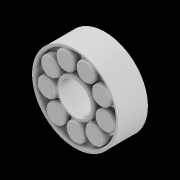
# Autodesk Inventor part: PIP-KL_parametriserad_02
Saved by Autodesk Inventor 2020 (Build 240168000, 168)
## iProperties
Created: 2020-11-21
Part Number: PIP-KL_parametriserad_02
Material: Generic
Document SubType Name: Modeling
Designer: Gottfrid
Density: 1 g/cm^3
Appearance: Default
Author: Gottfrid
Autodesk Inventor part; units mm, degrees
ref_plane "YZ Plane" through (0, 0, 0) normal (1, 0, 0) x (0, 1, 0)
ref_plane "XZ Plane" through (0, 0, 0) normal (0, 1, 0) x (-1, 0, 0)
ref_plane "XY Plane" through (0, 0, 0) normal (0, 0, 1) x (1, 0, 0)
sketch "Sketch1" plane through (0, 0, 0) normal (0, 0, 1) x (1, 0, 0)
  circle A0 centre (0, 0) radius 4
  circle A1 centre (0, 0) radius 4.75
  circle A2 centre (0, 0) radius 10
  circle A3 centre (0, 0) radius 10.75
  circle A4 centre (0, -7.375) radius 2.375
  dimension "d0" = 8
  dimension "d1" = 9.5
  dimension "d2" = 20
  dimension "d3" = 21.5
  dimension "d4" = 7.375
  dimension "d5" = 4.75
  constraints: 5 centre point, 4 coincident, 1 vertical alignment
  measures "d0" diameter of A0
  measures "d1" diameter of A1
  measures "d2" diameter of A2
  measures "d3" diameter of A3
  measures "d4" distance of A4.centre point (0, 0)
  measures "d5" diameter of A4
extrude "Extrusion1" add sketch "Sketch1" along normal blind 1.5 contours A0 | A1
extrude "Extrusion8" add sketch "Sketch1" along normal blind 1.5 contours A4
extrude "Extrusion9" add sketch "Sketch1" along normal blind 1.5 contours A3
sketch "Sketch17" plane through (0, 0, 1.5) normal (0, 0, 1) x (1, 0, 0)
  circle A0 centre (0, 0) radius 4.75 projected
extrude "Extrusion10" add sketch "Sketch17" along normal blind 1.5 draft 35
sketch "Sketch18" plane through (0, -7.375, 1.5) normal (0, 0, 1) x (1, 0, 0)
  circle A0 centre (0, 0) radius 2.375 projected
  point P0 (0, 7.375)
extrude "Extrusion11" add sketch "Sketch18" along normal blind 1.5 draft -35
sketch "Sketch19" plane through (0, 0, 1.5) normal (0, 0, 1) x (1, 0, 0)
  circle A0 centre (0, 0) radius 10 projected
  circle A1 centre (0, 0) radius 10.75 projected
extrude "Extrusion12" add sketch "Sketch19" along normal blind 1.5 draft 35
sketch "Sketch20" plane through (0, 0, 3) normal (0, 0, 1) x (1, 0, 0)
  circle A0 centre (0, 0) radius 5.8003 projected
extrude "Extrusion13" add sketch "Sketch20" along normal blind 0.75
sketch "Sketch21" plane through (0, -7.375, 3) normal (0, 0, 1) x (1, 0, 0)
  circle A0 centre (0, 0) radius 1.3247 projected
  point P0 (0, 7.375)
extrude "Extrusion14" add sketch "Sketch21" along normal blind 0.75
sketch "Sketch22" plane through (0, 0, 3) normal (0, 0, 1) x (1, 0, 0)
  circle A0 centre (0, 0) radius 8.9497 projected
  circle A1 centre (0, 0) radius 11.8003 projected
extrude "Extrusion15" add sketch "Sketch22" along normal blind 0.75
chamfer "Chamfer2" distance 0.3 angle 45 3 edges at (-10, 0, 0) (-2.375, -7.375, 0) (-4.75, 0, 0)
mirror "Mirror1" about plane through (0, 0, 3.75) normal (0, 0, 1) of "Extrusion13", "Extrusion10", "Extrusion1"
mirror "Mirror2" about plane through (0, -7.375, 3.75) normal (0, 0, 1) of "Extrusion8", "Extrusion11", "Extrusion14"
mirror "Mirror3" about plane through (0, 0, 3.75) normal (0, 0, 1) of "Extrusion9", "Extrusion12", "Extrusion15"
extrude "Extrusion16" cut sketch "Sketch1" along normal blind 99999 contours A0
extrude "Extrusion17" cut sketch "Sketch1" along normal blind 99999 contours A0 | A1 | A2 | A3 | A4 keep common part
chamfer "Chamfer3" distance 0.3 angle 45 3 edges at (-10, 0, 7.5) (-2.375, -7.375, 7.5) (-4.75, 0, 7.5)
pattern_circular "Circular Pattern2" count 9 over 360 about axis through (0, 0, 0) along (0, 0, 1) of "Extrusion8", "Extrusion11", "Extrusion14", "Mirror2"
chamfer "Chamfer4" distance 0.3 angle 45 14 edges at (-7.6754, 1.0583, 7.5) (-5.1994, 5.7443, 7.5) (-0.2906, 7.7425, 7.5) (4.7542, 6.1179, 7.5) (7.5744, 1.6307, 7.5) (6.8505, -3.6196, 7.5) (2.9212, -7.1762, 7.5) (2.9212, -7.1762, 0) (6.8505, -3.6196, 0) (7.5744, 1.6307, 0) (-0.2906, 7.7425, 0) (-5.1994, 5.7443, 0) (-7.6754, 1.0583, 0) (4.7542, 6.1179, 0)
equation "\"d0\" = 2 * r_inre"
equation "\"d1\" = 2 * r_inre + d_inreRing"
equation "\"d2\" = 2 * r_yttre"
equation "\"d3\" = 2 * r_yttre + d_yttreRing"
equation "\"d4\" = beräknad_avstånd_origo_till_rullkopp"
equation "\"d5\" = beräknad_diameter_rullkropp"
equation "\"d6\" = extrude_h1"
equation "\"d29\" = extrude_h1"
equation "\"d31\" = extrude_h1"
equation "\"d33\" = extrude_h1"
equation "\"d34\" = extrude_angle35"
equation "\"d35\" = extrude_h1"
equation "\"d36\" = -extrude_angle35"
equation "\"d37\" = extrude_h1"
equation "\"d38\" = extrude_angle35"
equation "\"d39\" = 0.5 * extrude_h1"
equation "\"d41\" = 0.5 * extrude_h1"
equation "\"d43\" = 0.5 * extrude_h1"
equation "\"d45\" = 0.2 * extrude_h1"
equation "\"d55\" = 0.2 * extrude_h1"
equation "\"d61\" = 0.2 * extrude_h1"
equation "\"r_inre\" = 4"
equation "\"d_inreRing\" = 1.5"
equation "\"d_yttreRing\" = 1.5"
equation "\"d_toleransMellanRullkroppOchRing\" = 0.25"
equation "\"extrude_h1\" = 1.5"
equation "\"extrude_angle35\" = 35deg"
equation "\"beräknad_diameter_rullkropp\" = r_yttre - 0.5 * d_inreRing - r_inre - 2 * d_toleransMellanRullkroppOchRing"
equation "\"beräknad_avstånd_origo_till_rullkopp\" = 0.5 * d_inreRing + r_inre + 0.5 * beräknad_diameter_rullkropp + d_toleransMellanRullkroppOchRing"
equation "\"r_yttre\" = 10"
body "Solid1"
